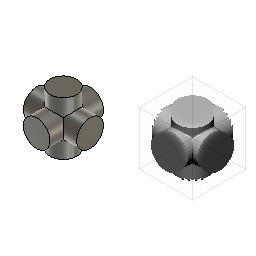
Custom Lattice (Autodesk Fusion 360 design; units mm, degrees)
Autodesk Fusion 360 part; units mm, degrees
sketch "Sketch1" plane through (0, 0, 0) normal (0, 0, 1) x (1, 0, 0)
  circle A0 centre (0, 0) radius 2.5
  dimension "d1" = 5
  constraint coincident A0.centre origin
  measures "d1" diameter of A0
extrude "Extrude1" add sketch "Sketch1" along normal mid plane 10 makes body 1
pattern_circular "C-Pattern1" count 2 over 90 about axis through (1.75, 0, 0) along (1, 0, 0) of bodies 1 makes body 2
pattern_circular "C-Pattern2" count 2 over 90 about axis through (0, 1.75, 0) along (0, 1, 0) of bodies 1 makes body 3
combine "Combine1" operation add target body 1 tool bodies 2 3
box "BoxPrimitive1" add length 10 width 10 height 10 placed x (0, -1, 0) y (1, 0, 0) z (0, 0, 1) at (15.427, 8.7372, 0) separate body makes body 4
